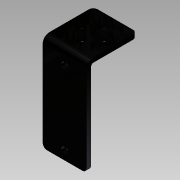
# Autodesk Inventor part: dudukanTPA
Saved by Autodesk Inventor 2015 SP1 (Build 190203100, 203)
## iProperties
Created: 2015-02-03
Part Number: dudukanTPA
Material: Generic
Document SubType Name: Modeling
Designer: Rafi Kurnia Putra
Density: 1 g/cm^3
Appearance: Smooth - Purple
Mass: 2.47397 g
Surface Area: 29.1677 cm^2
Volume: 2.47397 cm^3
Author: Rafi Kurnia Putra
Autodesk Inventor part; units mm, degrees
ref_plane "YZ Plane" through (0, 0, 0) normal (1, 0, 0) x (0, 1, 0)
ref_plane "XZ Plane" through (0, 0, 0) normal (0, 1, 0) x (-1, 0, 0)
ref_plane "XY Plane" through (0, 0, 0) normal (0, 0, 1) x (1, 0, 0)
sketch "Sketch1" plane through (0, 0, 0) normal (0, 0, 1) x (1, 0, 0)
  line L0 (-8, -20) -> (8, -20)
  line L1 (10, -18) -> (10, 20)
  line L2 (10, 20) -> (-10, 20)
  line L3 (-10, 20) -> (-10, -18)
  line L4 (-10, -20) -> (10, 20) construction
  line L5 (10, -20) -> (-10, 20) construction
  arc A0 (-10, -18) -> (-8, -20) centre (-8, -18) ccw
  arc A1 (8, -20) -> (10, -18) centre (8, -18) ccw
  point P0 (0, 0)
  dimension "d0" = 20
  dimension "d1" = 40
  dimension "d2" = 2
  constraints: 12 end point, 4 point on circle, 4 point on line, 4 tangent, 2 centre point, 2 midpoint, 2 parallel, 1 equal radius, 1 horizontal, 1 perpendicular
  measures "d0" distance of L2.end L1.end
  measures "d1" distance of L1.end L5.start
  measures "d2" radius of A0
extrude "Extrusion1" add sketch "Sketch1" along normal blind 2
sketch "Sketch2" plane through (0, 0, 0) normal (1, 0, 0) x (0, 1, 0)
  line L0 (20, 0) -> (20, 2) projected
  line L1 (20, 1) -> (21, 1)
  line L2 (23, 3) -> (23, 23)
  arc A0 (21, 1) -> (23, 3) centre (21, 3) ccw
  point P0 (0, 0)
  dimension "d5" = 2
  dimension "d8" = 20
  dimension "d9" = 1
  constraints: 4 end point, 2 point on circle, 2 tangent, 1 centre point, 1 horizontal, 1 midpoint, 1 perpendicular
  measures "d5" radius of A0
  measures "d8" distance of L2.start L2.end
  measures "d9" distance of L1.start L1.end
sketch "Sketch3" plane through (-10, 20, 0) normal (0, 1, 0) x (1, 0, 0)
  line L0 (0, 0) -> (20, 0) projected
  line L1 (0, 0) -> (0, -2) projected
  line L2 (20, -2) -> (0, -2) projected
  line L3 (20, 0) -> (20, -2) projected
  point P0 (10, 0)
sweep "Sweep1" add profiles "Sketch3" path "Sketch2" path curves L1 A0 L2
sketch "Sketch4" plane through (-10, 24, 3) normal (0, 1, 0) x (1, 0, 0)
  circle A0 centre (10, -5) radius 1.5
  circle A1 centre (10, -15) radius 1.5
  circle A2 centre (15, -10) radius 1.5
  circle A3 centre (5, -10) radius 1.5
  point P0 (10, -10)
  dimension "d10" = 3
  dimension "d11" = 3
  dimension "d12" = 3
  dimension "d13" = 3
  constraints: 4 centre point, 1 coincident
  measures "d10" diameter of A0
  measures "d11" diameter of A1
  measures "d12" diameter of A2
  measures "d13" diameter of A3
extrude "Extrusion2" cut sketch "Sketch4" against normal up to next
fillet "Fillet1" radius 2 2 edges at (10, 23, 23) (-10, 23, 23)
sketch "Sketch5" plane through (0, 0, 2) normal (0, 0, 1) x (1, 0, 0)
  circle A0 centre (0, -16.105) radius 1.5
  circle A1 centre (0, 17.225) radius 1.5
  point P0 (0, 0)
  dimension "d17" = 3
  dimension "d18" = 3
  dimension "d19" = 33.33
  constraints: 2 centre point
  measures "d17" diameter of A0
  measures "d18" diameter of A1
  measures "d19" distance of A1.centre A0.centre
extrude "Extrusion3" cut sketch "Sketch5" against normal through all
body "Solid1"
